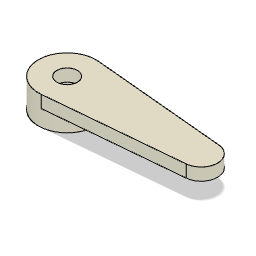
power_satellite_all (Autodesk Fusion 360 archive; units mm, degrees)
design "servo arm2"
Autodesk Fusion 360 part; units mm, degrees
sketch "Sketch1" plane through (0, 0, 0) normal (0, 1, 0) x (1, 0, 0)
  line L0 (0, 3.5) -> (0, -3.5) construction
  circle A0 centre (16.3288, 0) radius 2
  circle A1 centre (0, 0) radius 3.5
  line L1 (0.3215, 3.4852) -> (16.5126, 1.9915)
  line L2 (16.5126, -1.9915) -> (0.3215, -3.4852)
  line L3 (-3.3833, -0.8963) -> (18.1167, -0.8963) construction
  dimension "d2" = 7
  dimension "d12" = 21.5
  dimension "d13" = 4
  constraint vertical L0
  constraint midpoint A1.centre L0
  constraint coincident A1.centre origin
  constraint coincident L0.start A1
  constraint coincident A1 L1.start
  constraint coincident A0 L1.end
  constraint coincident A0 L2.start
  constraint coincident A1 L2.end
  constraint tangent A0 L1
  constraint tangent A1 L1
  constraint tangent A1 L2
  constraint tangent A0 L2
  constraint coincident A1 L3.start
  constraint coincident A0 L3.end
  constraint perpendicular L0 L3
  measures "d2" distance of L0.start L0.end
  measures "d12" distance of L3.start L3.end
  measures "d13" diameter of A0
extrude "Extrude1" add sketch "Sketch1" along normal blind 1.5
sketch "Sketch2" plane through (0, 0, 0) normal (0, -1, 0) x (1, 0, 0)
  arc A0 (0.3215, 3.4852) -> (0.3215, -3.4852) centre (0, 0) ccw
  line L0 (0.3215, -3.4852) -> (16.5126, -1.9915)
  arc A1 (16.5126, -1.9915) -> (16.5126, 1.9915) centre (16.3288, 0) ccw
  line L1 (16.5126, 1.9915) -> (0.3215, 3.4852)
  circle A2 centre (0, 0) radius 3.5
  circle A3 centre (0, 0) radius 2.95
  circle A4 centre (0, 0) radius 1.25
  dimension "d6" = 5.9
  dimension "d9" = 2.5
  constraint concentric A0 A2
  constraint concentric A2 A3
  constraint concentric A2 A4
  measures "d6" diameter of A3
  measures "d9" diameter of A4
extrude "Extrude2" add sketch "Sketch2" along normal blind 2 contours A0 A2
extrude "Extrude3" cut sketch "Sketch2" against normal blind 2 contours A4

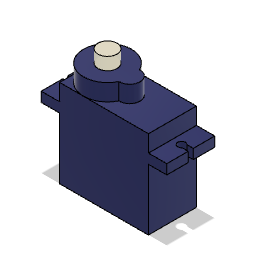
design "SG90"
Autodesk Fusion 360 part; units mm, degrees
sketch "Sketch1" plane through (0, 0, 0) normal (0, 0, 1) x (1, 0, 0)
  line L0 (0, 0) -> (22.8, 0)
  line L1 (22.8, 0) -> (22.8, 22.5)
  line L2 (22.8, 22.5) -> (0, 22.5)
  line L3 (0, 22.5) -> (0, 0)
  line L4 (7.397, 0) -> (7.397, 15.7) construction
  line L5 (-4.7, 15.7) -> (27.5, 15.7) construction
  line L6 (-4.7, 15.7) -> (0, 15.7)
  line L7 (22.8, 15.7) -> (27.5, 15.7)
  line L8 (-4.7, 15.7) -> (-4.7, 18.2)
  line L9 (-4.7, 18.2) -> (0, 18.2)
  line L10 (27.5, 15.7) -> (27.5, 18.2)
  line L11 (27.5, 18.2) -> (22.8, 18.2)
  dimension "d1" = 22.8
  dimension "d2" = 22.5
  dimension "d3" = 15.7
  dimension "d4" = 4.7
  dimension "d5" = 2.5
  constraint horizontal L0
  constraint vertical L1
  constraint horizontal L2
  constraint vertical L3
  constraint coincident L0.start L3.end
  constraint coincident L0 L4.start
  constraint perpendicular L0 L4
  constraint perpendicular L1 L5
  constraint coincident L4.end L5
  constraint coincident L5 L6.end
  constraint coincident L3 L6.end
  constraint coincident L1 L7.start
  constraint coincident L5 L7.start
  constraint equal L6 L7
  constraint perpendicular L6 L8
  constraint coincident L3 L9.end
  constraint perpendicular L3 L9
  constraint perpendicular L5 L10
  constraint equal L8 L10
  constraint coincident L1 L11.end
  constraint perpendicular L1 L11
  measures "d1" distance of L0.start L0.end
  measures "d2" distance of L0.start L2.end
  measures "d3" distance of L4.start L4.end
  measures "d4" distance of L5.start L6.end
  measures "d5" distance of L5.start L8.end
extrude "Extrude1" add sketch "Sketch1" along normal blind 12.3
sketch "Sketch2" plane through (0, 22.5, 0) normal (0, 1, 0) x (-1, 0, 0)
  line L0 (-22.8, 0) -> (0, 0)
  line L1 (0, 0) -> (0, 12.3)
  line L2 (0, 12.3) -> (-22.8, 12.3)
  line L3 (-22.8, 12.3) -> (-22.8, 0)
  circle A0 centre (-6.15, 6.15) radius 6.15
  line L4 (0, 6.15) -> (-14.5, 6.15)
  circle A1 centre (-11.85, 6.15) radius 2.65
  dimension "d8" = 14.5
  dimension "d9" = 5.3
  constraint tangent L0 A0
  constraint tangent L1 A0
  constraint tangent L2 A0
  constraint midpoint L1 L4.start
  constraint perpendicular L1 L4
  constraint coincident L4 A1.centre
  constraint coincident L4.end A1
  measures "d8" distance of L4.start L4.end
  measures "d9" diameter of A1
extrude "Extrude2" add sketch "Sketch2" along normal blind 4.3 contours A0 L4 A1 | A0 L4 A1 | A0 L4 A1 | A0 L4 A1 | A0 L4 A1 | A0 L4 A1
sketch "Sketch3" plane through (0, 26.8, 0) normal (0, 1, 0) x (-1, 0, 0)
  arc A0 (-11.7018, 3.5041) -> (-11.7018, 8.7959) centre (-6.15, 6.15) ccw
  arc A1 (-11.7018, 8.7959) -> (-11.7018, 3.5041) centre (-11.85, 6.15) ccw
  circle A2 centre (-6.15, 6.15) radius 2.45
  dimension "d12" = 4.9
  constraint concentric A0 A2
  measures "d12" diameter of A2
extrude "Extrude3" add sketch "Sketch3" along normal blind 3.2 contours A2
sketch "Sketch5" plane through (0, 18.2, 0) normal (0, 1, 0) x (-1, 0, 0)
  line L0 (0, 0) -> (4.7, 0)
  line L1 (4.7, 0) -> (4.7, 12.3)
  line L2 (4.7, 12.3) -> (0, 12.3)
  line L3 (0, 12.3) -> (0, 0)
  circle A0 centre (2.35, 6.15) radius 1
  line L4 (-27.5, 12.3) -> (-22.8, 0) construction
  circle A1 centre (-25.15, 6.15) radius 1
  line L5 (2.35, 5.5) -> (2.35, 6.8)
  line L6 (-25.15, 5.5) -> (-25.15, 6.8)
  line L7 (2.35, 5.5) -> (4.7, 5.5)
  line L8 (2.35, 6.8) -> (4.7, 6.8)
  line L9 (-25.15, 5.5) -> (-27.9, 5.5)
  line L10 (-25.15, 6.8) -> (-27.9, 6.8)
  line L11 (-27.9, 6.8) -> (-27.9, 5.5)
  dimension "d16" = 2
  dimension "d17" = 2
  dimension "d18" = 1.3
  dimension "d19" = 1.3
  constraint midpoint L4 A1.centre
  constraint vertical L5
  constraint midpoint A0.centre L5
  constraint vertical L6
  constraint midpoint A1.centre L6
  constraint coincident L1 L7.end
  constraint perpendicular L1 L7
  constraint coincident L1 L8.end
  constraint perpendicular L1 L8
  constraint perpendicular L6 L9
  constraint perpendicular L6 L10
  constraint perpendicular L9 L11
  measures "d16" diameter of A0
  measures "d17" diameter of A1
  measures "d18" distance of L5.start L5.end
  measures "d19" distance of L6.start L6.end
extrude "Extrude4" cut sketch "Sketch5" against normal blind 2.5 contours L1 A0 L7 L8 | A0 L5 L7 L8 | A0 L5 L7 L8 | A1 L6 L9 L10 | A1 L6 L9 L10 | A1 L9 L10 L11
